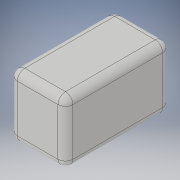
# Autodesk Inventor part: 7.3 Endhalterung Schiene
Saved by Autodesk Inventor 2018.3 (Build 223284000, 284)
## iProperties
Created: 2018-10-18
Part Number: 7.3 Endhalterung Schiene
Material: Generisch
Document SubType Name: Modeling
Designer: pgmadmin
Density: 1 g/cm^3
Appearance: Vorgabe
Author: pgmadmin
Autodesk Inventor part; units mm, degrees
ref_plane "YZ Plane" through (0, 0, 0) normal (1, 0, 0) x (0, 1, 0)
ref_plane "XZ Plane" through (0, 0, 0) normal (0, 1, 0) x (-1, 0, 0)
ref_plane "XY Plane" through (0, 0, 0) normal (0, 0, 1) x (1, 0, 0)
sketch "Skizze1" plane through (0, 0, 0) normal (0, 0, 1) x (1, 0, 0)
  line L0 (0, 0) -> (-22.3, 0)
  line L1 (-22.3, 0) -> (-22.3, 42)
  line L2 (-22.3, 42) -> (0, 42)
  line L3 (0, 42) -> (0, 0)
  line L4 (-19.3, 35) -> (-3, 35)
  line L5 (-3, 35) -> (-3, 33.4)
  line L6 (-3, 33.4) -> (-4.7, 33.4)
  line L7 (-4.7, 8.6) -> (-3, 8.6)
  line L8 (-3, 8.6) -> (-3, 7)
  line L9 (-3, 7) -> (-19.3, 7)
  line L10 (-19.3, 7) -> (-19.3, 35)
  line L11 (-4.7, 33.4) -> (-4.7, 8.6)
  line L12 (-11.15, 7) -> (-11.15, 0)
  line L13 (-11.15, 35) -> (-11.15, 42)
  dimension "d1" = 42
  dimension "d2" = 16.3
  dimension "d3" = 1.6
  dimension "d6" = 1.6
  dimension "d7" = 28
  dimension "d8" = 1.7
  dimension "d10" = 3
  dimension "d17" = 16.3
  dimension "d19" = 3
  constraints: 28 end point, 6 perpendicular, 4 midpoint, 2 horizontal, 2 parallel, 1 collinear, 1 vertical
  measures "d1" distance of L0.end L1.end
  measures "d2" distance of L4.start L4.end
  measures "d3" distance of L4.end L5.end
  measures "d6" distance of L7.end L8.end
  measures "d7" distance of L9.end L4.start
  measures "d8" distance of L6.end L5.end
  measures "d10" distance between parallel lines of L3 L5
  measures "d17" distance of L8.end L9.end
  measures "d19" distance between parallel lines of L1 L10
extrude "Extrusion1" add sketch "Skizze1" along normal blind 20 contours L0 L12 L9 L8 L7 L11 L6 L5 L4 L13 L2 L3 | L0 L1 L2 L13 L4 L10 L9 L12
sketch "Skizze2" plane through (0, 0, 20) normal (0, 0, 1) x (1, 0, 0)
  line L0 (0, 42) -> (-22.3, 42) projected
  line L1 (-22.3, 42) -> (0, 42)
  line L2 (0, 42) -> (0, 0)
  line L3 (0, 0) -> (-22.3, 0)
  line L4 (-22.3, 0) -> (-22.3, 42)
  constraints: 8 end point, 2 parallel, 1 horizontal, 1 perpendicular
extrude "Extrusion2" add sketch "Skizze2" along normal blind 5
fillet "Rundung1" radius 3 12 edges at (-11.15, 0, 0) (-22.3, 21, 0) (0, 21, 0) (-11.15, 42, 0) (0, 21, 25) (0, 0, 12.5) (-11.15, 0, 25) (-22.3, 0, 12.5) (-22.3, 21, 25) (-11.15, 42, 25) (0, 42, 12.5) (-22.3, 42, 12.5)
